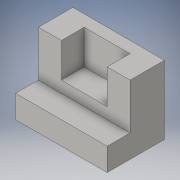
# Autodesk Inventor part: Figure 7_27_6
Saved by Autodesk Inventor 2016 (Build 200138000, 138)
## iProperties
Created: 2016-07-18
Part Number: Figure 7_27_6
Material: Generic
Document SubType Name: Modeling
Designer: cfkguest
Density: 1 g/cm^3
Appearance: Default
Author: cfkguest
Autodesk Inventor part; units mm, degrees
ref_plane "YZ Plane" through (0, 0, 0) normal (1, 0, 0) x (0, 1, 0)
ref_plane "XZ Plane" through (0, 0, 0) normal (0, 1, 0) x (-1, 0, 0)
ref_plane "XY Plane" through (0, 0, 0) normal (0, 0, 1) x (1, 0, 0)
sketch "Sketch1" plane through (0, 0, 0) normal (0, 0, 1) x (1, 0, 0)
  line L0 (-33.6112, 18.3384) -> (17.1888, 18.3384)
  line L1 (17.1888, 18.3384) -> (17.1888, -19.7616)
  line L2 (17.1888, -19.7616) -> (-33.6112, -19.7616)
  line L3 (-33.6112, -19.7616) -> (-33.6112, 18.3384)
  point P0 (0, 0)
  dimension "d0" = 50.8
  dimension "d1" = 38.1
  constraints: 8 end point, 2 parallel, 1 horizontal, 1 perpendicular
  measures "d0" distance of L0.start L0.end
  measures "d1" distance of L0.end L1.end
extrude "Extrusion1" add sketch "Sketch1" along normal blind 31.75
sketch "Sketch2" plane through (0, 0, 31.75) normal (0, 0, 1) x (1, 0, 0)
  line L0 (17.1888, 18.3384) -> (-33.6112, 18.3384) projected
  line L1 (17.1888, -19.7616) -> (17.1888, 18.3384) projected
  line L2 (-33.6112, 18.3384) -> (17.1888, 18.3384)
  line L3 (17.1888, 18.3384) -> (17.1888, -7.0616)
  line L4 (17.1888, -7.0616) -> (-33.6112, -7.0616)
  line L5 (-33.6112, -7.0616) -> (-33.6112, 18.3384)
  line L6 (17.1888, -19.7616) -> (-33.6112, -19.7616) projected
  point P0 (0, 0)
  dimension "d4" = 12.7
  constraints: 8 end point, 2 parallel, 1 horizontal, 1 perpendicular, 1 point on line
  measures "d4" distance between parallel lines of L6 L4
extrude "Extrusion2" cut sketch "Sketch2" against normal blind 12.7
sketch "Sketch3" plane through (0, 0, 19.05) normal (0, 0, 1) x (1, 0, 0)
  line L0 (-33.6112, 18.3384) -> (17.1888, 18.3384) projected
  line L1 (-20.9112, 18.3384) -> (4.4888, 18.3384)
  line L2 (4.4888, 18.3384) -> (4.4888, -0.7116)
  line L3 (4.4888, -0.7116) -> (-20.9112, -0.7116)
  line L4 (-20.9112, -0.7116) -> (-20.9112, 18.3384)
  line L5 (17.1888, 18.3384) -> (17.1888, -7.0616) projected
  point P0 (0, 0)
  dimension "d7" = 25.4
  dimension "d8" = 12.7
  dimension "d9" = 19.05
  constraints: 8 end point, 2 parallel, 1 horizontal, 1 perpendicular, 1 point on line
  measures "d7" distance of L2.end L3.end
  measures "d8" distance between parallel lines of L5 L2
  measures "d9" distance of L3.end L1.start
extrude "Extrusion3" cut sketch "Sketch3" against normal blind 12.7
body "Solid1"
